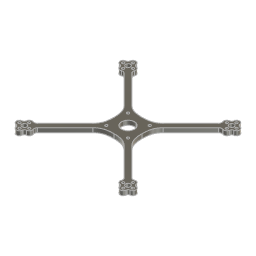
3 Zoll Frame v1 (Autodesk Fusion 360 design; units mm, degrees)
Autodesk Fusion 360 part; units mm, degrees
sketch "Skizze1" plane through (0, 0, 0) normal (0, 0, 1) x (1, 0, 0)
  line L0 (-47.9408, 47.9408) -> (47.9408, 47.9408) construction
  line L1 (47.9408, 47.9408) -> (47.9408, -47.9408) construction
  line L2 (47.9408, -47.9408) -> (-47.9408, -47.9408) construction
  line L3 (-47.9408, -47.9408) -> (-47.9408, 47.9408) construction
  line L4 (-47.9408, 47.9408) -> (47.9408, -47.9408) construction
  line L5 (47.9408, 47.9408) -> (-47.9408, -47.9408) construction
  circle A0 centre (-47.9408, 47.9408) radius 38.1 construction
  circle A1 centre (-47.9408, -47.9408) radius 38.1 construction
  circle A2 centre (47.9408, -47.9408) radius 38.1 construction
  circle A3 centre (47.9408, 47.9408) radius 38.1 construction
  line L6 (-21, 21) -> (21, 21) construction
  line L7 (21, 21) -> (21, -21) construction
  line L8 (21, -21) -> (-21, -21) construction
  line L9 (-21, -21) -> (-21, 21) construction
  line L10 (-21, 21) -> (21, -21) construction
  line L11 (21, 21) -> (-21, -21) construction
  circle A4 centre (47.9408, 47.9408) radius 2.25
  circle A5 centre (43.4408, 47.9408) radius 1.1
  circle A6 centre (47.9408, 43.4408) radius 1.1
  circle A7 centre (52.4408, 47.9408) radius 1.1
  circle A8 centre (47.9408, 52.4408) radius 1.1
  circle A9 centre (47.9408, 47.9408) radius 4.5 construction
  line L12 (45.1158, 52.4408) -> (45.1158, 43.4408)
  arc A10 (45.1158, 43.4408) -> (50.7658, 43.4408) centre (47.9408, 43.4408) ccw
  line L13 (50.7658, 43.4408) -> (50.7658, 52.4408)
  arc A11 (50.7658, 52.4408) -> (45.1158, 52.4408) centre (47.9408, 52.4408) ccw
  line L14 (47.9408, 52.4408) -> (47.9408, 43.4408) construction
  line L15 (43.4408, 45.1158) -> (52.4408, 45.1158)
  arc A12 (52.4408, 45.1158) -> (52.4408, 50.7658) centre (52.4408, 47.9408) ccw
  line L16 (52.4408, 50.7658) -> (43.4408, 50.7658)
  arc A13 (43.4408, 50.7658) -> (43.4408, 45.1158) centre (43.4408, 47.9408) ccw
  line L17 (43.4408, 47.9408) -> (52.4408, 47.9408) construction
  circle A14 centre (47.9408, 52.4408) radius 1.825 construction
  line L18 (-10, 10) -> (10, 10) construction
  line L19 (10, 10) -> (10, -10) construction
  line L20 (10, -10) -> (-10, -10) construction
  line L21 (-10, -10) -> (-10, 10) construction
  line L22 (-10, 10) -> (10, -10) construction
  line L23 (10, 10) -> (-10, -10) construction
  circle A15 centre (10, 10) radius 1.1
  circle A16 centre (0, 0) radius 6
  line L24 (-18, 18) -> (18, 18) construction
  line L25 (18, 18) -> (18, -18) construction
  line L26 (18, -18) -> (-18, -18) construction
  line L27 (-18, -18) -> (-18, 18) construction
  line L28 (-18, 18) -> (18, -18) construction
  line L29 (18, 18) -> (-18, -18) construction
  line L30 (-47.9408, 47.9408) -> (47.9408, -47.9408) construction
  line L31 (-21, -21) -> (-21, 21) construction
  line L32 (-47.9408, 47.9408) -> (47.9408, 47.9408) construction
  circle A17 centre (-47.9408, 47.9408) radius 38.1 construction
  line L33 (-21, 21) -> (21, -21) construction
  line L34 (-21, 21) -> (21, 21) construction
  line L35 (-47.9408, -47.9408) -> (-47.9408, 47.9408) construction
  line L36 (-47.9408, -47.9408) -> (47.9408, 47.9408) construction
  line L37 (21, -21) -> (-21, -21) construction
  line L38 (-47.9408, -47.9408) -> (-47.9408, 47.9408) construction
  circle A18 centre (-47.9408, -47.9408) radius 38.1 construction
  line L39 (-21, -21) -> (21, 21) construction
  line L40 (-21, -21) -> (-21, 21) construction
  line L41 (47.9408, -47.9408) -> (-47.9408, -47.9408) construction
  line L42 (47.9408, -47.9408) -> (-47.9408, 47.9408) construction
  line L43 (21, 21) -> (21, -21) construction
  line L44 (47.9408, -47.9408) -> (-47.9408, -47.9408) construction
  circle A19 centre (47.9408, -47.9408) radius 38.1 construction
  line L45 (21, -21) -> (-21, 21) construction
  line L46 (21, -21) -> (-21, -21) construction
  line L47 (47.9408, 47.9408) -> (47.9408, -47.9408) construction
  line L48 (14.4645, 18) -> (41.9845, 45.52)
  line L49 (18, 14.4645) -> (45.52, 41.9845)
  line L50 (0, 0) -> (0, 13)
  line L51 (0, 0) -> (13, 0)
  spline S0 degree 5 poles (18, 14.4645) (17.446, 13.9105) (16.4408, 12.7983) (15.2412, 11.1172) (14.1733, 8.8515) (13.4312, 5.9753) (13.133, 3.6274) (13.0242, 1.83) (13, 0.6131) (13, 0) knots 0 0 0 0 0 0 0.2 0.4 0.6 0.8 1 1 1 1 1 1
  spline S1 degree 5 poles (0, 13) (0.6107, 13) (1.8239, 13.0245) (3.6195, 13.1347) (5.9707, 13.4361) (8.8547, 14.1818) (11.124, 15.2498) (12.8037, 16.4466) (13.9127, 17.4482) (14.4645, 18) knots 0 0 0 0 0 0 0.2 0.4 0.6 0.8 1 1 1 1 1 1
  line L52 (18.8839, 15.3483) -> (17.1161, 13.5806)
  line L53 (13.5806, 17.1161) -> (15.3483, 18.8839)
  line L54 (-1, 13) -> (1, 13)
  line L55 (13, 1) -> (13, -1)
  line L56 (0, 0) -> (55.2658, 0)
  line L57 (55.2658, 0) -> (55.2658, 55.2658) construction
  line L58 (55.2658, 55.2658) -> (0, 55.2658) construction
  line L59 (0, 55.2658) -> (0, 0)
  dimension "d1" = 76.2
  dimension "d2" = 42
  dimension "d3" = 4.5
  dimension "d4" = 2.2
  dimension "d5" = 9
  dimension "d6" = 3.65
  dimension "d7" = 1
  dimension "d8" = 20
  dimension "d9" = 2.2
  dimension "d10" = 12
  dimension "d11" = 8
  dimension "d22" = 5
  dimension "d25" = 2.5
  dimension "d26" = 2
  dimension "d36" = 55.2658
  dimension "d37" = 5
  constraint horizontal L0
  constraint perpendicular L0 L1
  constraint parallel L0 L2
  constraint parallel L1 L3
  constraint coincident L4 A16.centre
  constraint coincident L5 A16.centre
  constraint coincident A16.centre L50.start
  constraint coincident L0.start L3.end
  constraint coincident L2.end L3.start
  constraint coincident L1.end L2.start
  constraint coincident L0.end L1.start
  constraint equal A0 A3
  constraint equal A1 A2
  constraint equal A1 A3
  constraint equal L0 L1
  constraint horizontal L6
  constraint perpendicular L6 L7
  constraint parallel L6 L8
  constraint parallel L7 L9
  constraint coincident L10 A16.centre
  constraint coincident L11 A16.centre
  constraint equal L6 L7
  constraint coincident A0 L6.start
  constraint concentric A3 A4
  constraint coincident L0 A5.centre
  constraint coincident L1 A6.centre
  constraint horizontal A5.centre A7.centre
  constraint vertical A6.centre A8.centre
  constraint equal A5 A8
  constraint equal A6 A7
  constraint equal A5 A6
  constraint concentric A3 A9
  constraint coincident A8.centre A9
  constraint coincident A5.centre A9
  constraint coincident A6.centre A9
  constraint coincident A7.centre A9
  constraint tangent L12 A10
  constraint tangent A10 L13
  constraint parallel L12 L13
  constraint tangent L13 A11
  constraint tangent L12 A11
  constraint coincident A6.centre A10.centre
  constraint parallel L1 L14
  constraint coincident A8.centre A11.centre
  constraint tangent L15 A12
  constraint tangent A12 L16
  constraint parallel L15 L16
  constraint tangent L16 A13
  constraint tangent L15 A13
  constraint coincident A7.centre A12.centre
  constraint parallel L0 L17
  constraint coincident A5.centre A13.centre
  constraint equal A11 A13
  constraint concentric A11 A14
  constraint horizontal L18
  constraint perpendicular L18 L19
  constraint parallel L18 L20
  constraint parallel L19 L21
  constraint coincident L22 A16.centre
  constraint coincident L23 A16.centre
  constraint coincident L4 L18.start
  constraint coincident L18.end L19.start
  constraint horizontal L24
  constraint perpendicular L24 L25
  constraint parallel L24 L26
  constraint parallel L25 L27
  constraint coincident L28 A16.centre
  constraint coincident L29 A16.centre
  constraint coincident L10 L24.start
  constraint coincident A13 L48.end
  constraint coincident A10 L49.end
  constraint symmetric L5 L48 L49
  constraint parallel L48 L49
  constraint coincident L24 L48.start
  constraint coincident L25 L49.start
  constraint perpendicular L24 L50
  constraint perpendicular L19 L51
  constraint midpoint L49.start L52
  constraint collinear L49 L52
  constraint midpoint L48.start L53
  constraint collinear L48 L53
  constraint equal L52 L53
  constraint midpoint L50.end L54
  constraint perpendicular L50 L54
  constraint midpoint L51.end L55
  constraint perpendicular L51 L55
  constraint equal L54 L55
  constraint equal L50 L51
  constraint horizontal L56
  constraint vertical L57
  constraint horizontal L58
  constraint vertical L59
  constraint tangent A12 L57
  constraint tangent A11 L58
  measures "d1" diameter of A0
  measures "d2" distance of L6.start L6.end
  measures "d3" diameter of A4
  measures "d4" diameter of A8
  measures "d5" diameter of A9
  measures "d6" diameter of A14
  measures "d7" distance of A11 A14
  measures "d8" distance of L18.start L18.end
  measures "d9" diameter of A15
  measures "d10" diameter of A16
  measures "d11" distance of L18.start L24
  measures "d22" distance of L48 L49
  measures "d25" distance of L53.start L53.end
  measures "d26" distance of L54.start L54.end
  measures "d36" distance of L56.end L57.end
  measures "d37" distance of L24 L50.end
extrude "Extrusion2" add sketch "Skizze1" along normal blind 4 contours L12 L13 A11 L16 | L12 L13 L15 L16 | L12 L15 L16 A13 | L12 A10 L13 L15 | L12 A10 L15 A13 A16 L48 L49 L50 L51 S0 S1 L52 L53 L56 L59 | L13 L15 A12 L16 makes body 1
fillet "Abrundung2" radius 3 2 edges at (45.52, 41.9845, 2) (41.9845, 45.52, 2) on bodies 1
fillet "Abrundung3" radius 2 3 edges at (50.7658, 45.1158, 2) (50.7658, 50.7658, 2) (45.1158, 50.7658, 2) on bodies 1
pattern_circular "C-Anordnung1" count 4 over 360 about axis through (0, 0, 1.75) along (0, 0, 1) of bodies 1 makes body 2 at (-32.7629, 33.9414, 4) makes body 3 at (-33.9414, -32.7629, 4) makes body 4 at (32.7629, -33.9414, 4)
combine "Kombinieren1" operation add target body 2 tool bodies 1 3 4
